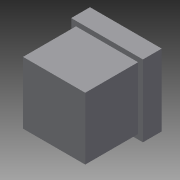
# Autodesk Inventor part: RFCoupler
Saved by Autodesk Inventor 2014 (Build 180170000, 170)
## iProperties
Created: 2015-03-25
Part Number: RFCoupler
Material: Generic
Document SubType Name: Modeling
Designer: Owner
Density: 1 g/cm^3
Appearance: Gray
Author: Owner
Autodesk Inventor part; units mm, degrees
ref_plane "YZ Plane" through (0, 0, 0) normal (1, 0, 0) x (0, 1, 0)
ref_plane "XZ Plane" through (0, 0, 0) normal (0, 1, 0) x (-1, 0, 0)
ref_plane "XY Plane" through (0, 0, 0) normal (0, 0, 1) x (1, 0, 0)
sketch "Sketch1" plane through (0, 0, 0) normal (0, 0, 1) x (1, 0, 0)
  line L0 (11.4609, 7.1382) -> (15.2709, 7.1382)
  line L1 (15.2709, 7.1382) -> (15.2709, 3.3282)
  line L2 (15.2709, 3.3282) -> (11.4609, 3.3282)
  line L3 (11.4609, 3.3282) -> (11.4609, 7.1382)
  point P0 (0, 0)
  dimension "d0" = 3.81
  dimension "d1" = 3.81
  constraints: 8 end point, 2 parallel, 1 horizontal, 1 perpendicular
  measures "d0" distance of L0.start L0.end
  measures "d1" distance of L0.end L1.end
extrude "Extrusion1" add sketch "Sketch1" along normal blind 1
sketch "Sketch2" plane through (0, 0, 1) normal (0, 0, 1) x (1, 0, 0)
  line L0 (15.2709, 7.1382) -> (11.4609, 7.1382) projected
  line L1 (15.2709, 3.3282) -> (15.2709, 7.1382) projected
  line L2 (11.7149, 6.8842) -> (15.0169, 6.8842)
  line L3 (15.0169, 6.8842) -> (15.0169, 3.5822)
  line L4 (15.0169, 3.5822) -> (11.7149, 3.5822)
  line L5 (11.7149, 3.5822) -> (11.7149, 6.8842)
  line L6 (11.4609, 7.1382) -> (11.4609, 3.3282) projected
  line L7 (11.4609, 3.3282) -> (15.2709, 3.3282) projected
  point P0 (0, 0)
  dimension "d6" = 0.254
  dimension "d7" = 0.254
  dimension "d10" = 0.254
  dimension "d11" = 0.254
  constraints: 8 end point, 2 parallel, 1 horizontal, 1 perpendicular
  measures "d6" distance between parallel lines of L0 L2
  measures "d7" distance between parallel lines of L1 L3
  measures "d10" distance between parallel lines of L6 L5
  measures "d11" distance between parallel lines of L7 L4
extrude "Extrusion2" add sketch "Sketch2" along normal blind 2.81 contours L2 L3 L4 L5
body "Solid1"
